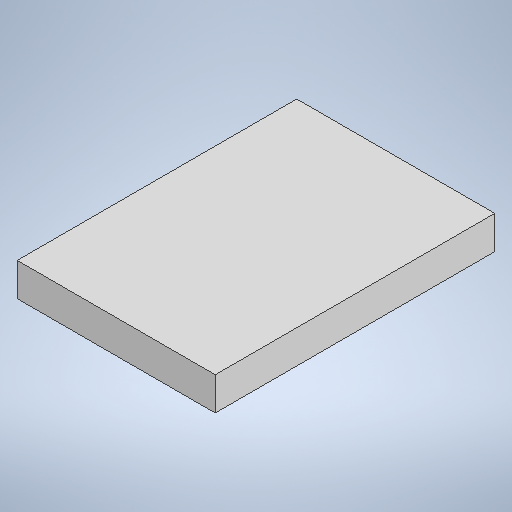
# Autodesk Inventor part: UWB
Saved by Autodesk Inventor 2025.2 (Build 292293000, 293)
## iProperties
Created: 2026-03-13
Part Number: UWB
Material: Genérico
Document SubType Name: Modeling
Designer: Periscopio
Density: 1 g/cm^3
Appearance: Valor por defecto
Author: Periscopio
Autodesk Inventor part; units mm, degrees
ref_plane "YZ Plane" through (0, 0, 0) normal (1, 0, 0) x (0, 1, 0)
ref_plane "XZ Plane" through (0, 0, 0) normal (0, 1, 0) x (-1, 0, 0)
ref_plane "XY Plane" through (0, 0, 0) normal (0, 0, 1) x (1, 0, 0)
sketch "Boceto1" plane through (0, 0, 0) normal (0, 1, 0) x (-1, 0, 0)
  line L0 (9.565, -13.5) -> (-9.565, -13.5)
  line L1 (-9.565, -13.5) -> (-9.565, 13.5)
  line L2 (-9.565, 13.5) -> (9.565, 13.5)
  line L3 (9.565, 13.5) -> (9.565, -13.5)
  line L4 (9.565, -13.5) -> (-9.565, 13.5) construction
  line L5 (-9.565, -13.5) -> (9.565, 13.5) construction
  point P0 (0, 0)
  point P1 (0, 0)
  dimension "d0" = 19.13
  dimension "d1" = 27
  constraints: 12 end point, 2 midpoint, 2 parallel, 1 coincident, 1 horizontal, 1 perpendicular
  measures "d0" distance of L1.end L2.end
  measures "d1" distance of L0.end L1.end
extrude "Extrusión1" add sketch "Boceto1" along normal blind 3.2
